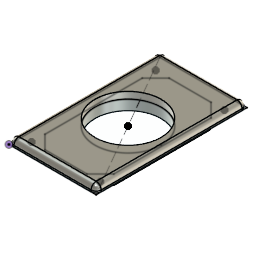
JD19.5mm_buttonholder v1 (Autodesk Fusion 360 design; units mm, degrees)
Autodesk Fusion 360 part; units mm, degrees
sketch "Sketch1" plane through (0, 0, 0) normal (0, 0, 1) x (1, 0, 0)
  line L0 (0, 0) -> (26, 0)
  line L1 (26, 0) -> (26, 45)
  line L2 (26, 45) -> (0, 45)
  line L3 (0, 45) -> (0, 0)
  line L4 (0, 45) -> (26, 0) construction
  circle A0 centre (13, 22.5) radius 9.85
  line L5 (6.75, 4) -> (19.25, 4)
  line L6 (23.25, 8) -> (23.25, 37)
  line L7 (19.25, 41) -> (6.75, 41)
  line L8 (2.75, 37) -> (2.75, 8)
  line L9 (6.75, 41) -> (2.75, 37)
  line L10 (23.25, 37) -> (19.25, 41)
  line L11 (6.75, 4) -> (2.75, 8)
  line L12 (23.25, 8) -> (19.25, 4)
  point P0 (2.75, 4)
  point P1 (23.25, 4)
  point P2 (23.25, 41)
  point P3 (2.75, 41)
  dimension "d1" = 19.7
  dimension "d2" = 26
  dimension "d3" = 45
  dimension "d4" = 20.5
  dimension "d5" = 2.75
  dimension "d6" = 4
  dimension "d7" = 37
  dimension "d8" = 4
  dimension "d9" = 4
  dimension "d10" = 4
  dimension "d11" = 4
  dimension "d12" = 4
  dimension "d13" = 4
  dimension "d14" = 4
  dimension "d15" = 4
  constraint horizontal L0
  constraint vertical L1
  constraint horizontal L2
  constraint vertical L3
  constraint coincident L0.start L3.end
  constraint midpoint L4 A0.centre
  constraint horizontal L5
  constraint vertical L6
  constraint horizontal L7
  constraint vertical L8
  constraint coincident P3 L7
  constraint coincident P3 L8
  constraint coincident P2 L6
  constraint coincident P2 L7
  constraint coincident P0 L5
  constraint coincident P0 L8
  constraint coincident P1 L6
  constraint coincident P1 L5
  measures "d1" diameter of A0
  measures "d2" distance of L0.start L0.end
  measures "d3" distance of L0.start L2.end
  measures "d4" distance of P0 P1
  measures "d5" distance of L3 L8
  measures "d6" distance of L0 L5
  measures "d7" distance of P0 P3
  measures "d8" distance of P3 L7.end
  measures "d9" distance of P3 L8.start
  measures "d10" distance of P2 L6.end
  measures "d11" distance of P2 L7.start
  measures "d12" distance of P0 L5.start
  measures "d13" distance of P0 L8.end
  measures "d14" distance of P1 L6.start
  measures "d15" distance of P1 L5.end
extrude "Extrude1" add sketch "Sketch1" along normal blind 2 contours L0 L1 L2 L3 | L5 L6 L7 L8 L9 L10 L11 L12
extrude "Extrude2" add sketch "Sketch1" against normal blind 3 contours L5 L6 L7 L8 L9 L10 L11 L12
fillet "Fillet1" radius 1.5 16 edges at (26, 0, 1) (0, 0, 1) (0, 45, 1) (26, 45, 1) (6.75, 41, -1.5) (2.75, 37, -1.5) (19.25, 41, -1.5) (23.25, 37, -1.5) (23.25, 8, -1.5) (19.25, 4, -1.5) (6.75, 4, -1.5) (2.75, 8, -1.5) (13, 45, 2) (0, 22.5, 2) (13, 0, 2) (26, 22.5, 2)
equation "d5 = ( d2 - d4 ) / 2"
equation "d6 = ( d3 - d7 ) / 2"
equation "d9 = d8"
equation "d10 = d8"
equation "d11 = d10"
equation "d12 = d8"
equation "d13 = d12"
equation "d14 = d8"
equation "d15 = d14"
